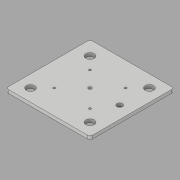
# Autodesk Inventor part: E_base2
Saved by Autodesk Inventor 2019 (Build 230136000, 136)
## iProperties
Created: 2021-11-01
Part Number: E_base2
Material: Generic
Document SubType Name: Modeling
Designer: Mohamed
Density: 1 g/cm^3
Appearance: Default
Author: Mohamed
Autodesk Inventor part; units mm, degrees
ref_plane "YZ Plane" through (0, 0, 0) normal (1, 0, 0) x (0, 1, 0)
ref_plane "XZ Plane" through (0, 0, 0) normal (0, 1, 0) x (-1, 0, 0)
ref_plane "XY Plane" through (0, 0, 0) normal (0, 0, 1) x (1, 0, 0)
sketch "Sketch1" plane through (0, 0, 0) normal (0, 1, 0) x (-1, 0, 0)
  line L0 (5, 0) -> (145, 0)
  line L1 (150, -5) -> (150, -145)
  line L2 (145, -150) -> (5, -150)
  line L3 (0, -145) -> (0, -5)
  arc A0 (150, -5) -> (145, 0) centre (145, -5) ccw
  arc A1 (150, -5) -> (145, 0) centre (145, -5) ccw
  arc A2 (145, -150) -> (150, -145) centre (145, -145) ccw
  arc A3 (5, 0) -> (0, -5) centre (5, -5) ccw
  arc A4 (0, -145) -> (5, -150) centre (5, -145) ccw
  circle A5 centre (128.033, -21.967) radius 7.5
  circle A6 centre (124.4975, -124.4975) radius 7.5
  circle A7 centre (21.967, -128.033) radius 7.5
  circle A8 centre (21.967, -21.967) radius 7.5
  circle A9 centre (21.967, -75) radius 5
  point P0 (150, -150)
  point P1 (150, 0)
  point P2 (0, -150)
  dimension "d12" = 150
  dimension "d13" = 150
  dimension "d22" = 5
  dimension "d23" = 5
  dimension "d28" = 15
  dimension "d29" = 15
  dimension "d30" = 15
  dimension "d31" = 15
  dimension "d32" = 10
  constraints: 10 centre point, 10 point on circle, 10 tangent, 8 end point, 8 point on line, 3 equal radius, 2 parallel, 1 horizontal, 1 perpendicular
  measures "d12" distance of point (150, -150) point (0, -150)
  measures "d13" distance of point (150, 0) point (150, -150)
  measures "d22" radius of A0
  measures "d23" radius of A2
  measures "d28" diameter of A5
  measures "d29" diameter of A6
  measures "d30" diameter of A7
  measures "d31" diameter of A8
  measures "d32" diameter of A9
extrude "Extrusion1" add sketch "Sketch1" along normal blind 6
sketch "Sketch2" plane through (0, 6, 0) normal (0, 1, 0) x (1, 0, 0)
  arc A0 (-5, 0) -> (0, 5) centre (-5, 5) ccw projected
  arc A1 (-145, 150) -> (-150, 145) centre (-145, 145) ccw projected
  arc A2 (-150, 5) -> (-145, 0) centre (-145, 5) ccw projected
  circle A3 centre (-21.967, 128.033) radius 7.5 projected
  circle A4 centre (-128.033, 21.967) radius 7.5 projected
  circle A5 centre (-124.4975, 124.4975) radius 7.5 projected
  circle A6 centre (-106.8198, 43.1802) radius 2
  circle A7 centre (-102.8482, 102.8482) radius 2
  circle A8 centre (-43.1802, 43.1802) radius 2
  circle A9 centre (-43.1802, 106.8198) radius 2
  circle A10 centre (-75, 75) radius 3
  point P0 (0, 0)
  dimension "d39" = 4
  dimension "d40" = 4
  dimension "d41" = 4
  dimension "d42" = 4
  dimension "d43" = 6
  constraints: 5 centre point
  measures "d39" diameter of A6
  measures "d40" diameter of A7
  measures "d41" diameter of A8
  measures "d42" diameter of A9
  measures "d43" diameter of A10
extrude "Extrusion2" cut sketch "Sketch2" against normal blind 6 contours A6 | A7 | A8 | A9 | A10
body "Solid1"
